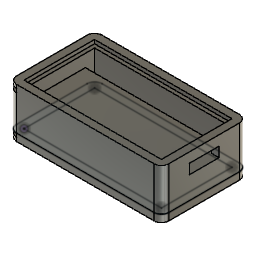
ESP 32 Case (Autodesk Fusion 360 design; units mm, degrees)
Autodesk Fusion 360 part; units mm, degrees
sketch "Sketch1" plane through (0, 0, 0) normal (0, 0, 1) x (1, 0, 0)
  line L0 (0, 0) -> (55.5, 0)
  line L1 (55.5, 0) -> (55.5, 28.5)
  line L2 (55.5, 28.5) -> (0, 28.5)
  line L3 (0, 28.5) -> (0, 0)
  line L4 (0, -3) -> (55.5, -3)
  line L5 (58.5, 0) -> (58.5, 28.5)
  line L6 (55.5, 31.5) -> (0, 31.5)
  line L7 (-3, 28.5) -> (-3, 0)
  arc A0 (58.5, 28.5) -> (55.5, 31.5) centre (55.5, 28.5) ccw
  arc A1 (55.5, -3) -> (58.5, 0) centre (55.5, 0) ccw
  arc A2 (-3, 0) -> (0, -3) centre (0, 0) ccw
  arc A3 (0, 31.5) -> (-3, 28.5) centre (0, 28.5) ccw
  dimension "d1" = 55.5
  dimension "d2" = 28.5
  dimension "d4" = 3
  dimension "d5" = 3
  dimension "d6" = 3
  dimension "d7" = 3
  constraint horizontal L0
  constraint vertical L1
  constraint horizontal L2
  constraint vertical L3
  constraint coincident L0.start L3.end
  constraint tangent L5 A0
  constraint tangent L6 A0
  constraint tangent L4 A1
  constraint tangent L5 A1
  constraint tangent L7 A2
  constraint tangent L4 A2
  constraint tangent L6 A3
  constraint tangent L7 A3
  measures "d1" distance of L0.start L0.end
  measures "d2" distance of L0.end L1.end
  measures "d4" radius of A0
  measures "d5" radius of A1
  measures "d6" radius of A2
  measures "d7" radius of A3
extrude "Extrude1" add sketch "Sketch1" along normal blind 12.7 makes body 1
extrude "Extrude2" add sketch "Sketch1" along normal blind 14 separate body makes body 2
sketch "Sketch3" plane through (0, 0, 0) normal (1, 0, 0) x (0, 1, 0)
  line L0 (0, 0) -> (28.5, 0)
  line L1 (28.5, 0) -> (28.5, 14)
  line L2 (28.5, 14) -> (0, 14)
  line L3 (0, 14) -> (0, 0)
  line L4 (13, 9) -> (28.5, 9)
  line L5 (28.5, 9) -> (28.5, 7)
  line L6 (28.5, 7) -> (13, 7)
  line L7 (13, 7) -> (0, 7)
  line L8 (0, 7) -> (0, 9)
  line L9 (0, 9) -> (13, 9)
  line L10 (3.75, 9) -> (3.75, 7)
  line L11 (24.75, 9) -> (24.75, 7)
  dimension "d13" = 5
  dimension "d14" = 5
  dimension "d15" = 2
  dimension "d16" = 21
  dimension "d17" = 3.75
  constraint horizontal L4
  constraint vertical L5
  constraint horizontal L6
  constraint coincident L1 L5.end
  constraint horizontal L7
  constraint vertical L8
  constraint horizontal L9
  constraint coincident L3 L8.end
  constraint coincident L9 L10.start
  constraint coincident L7 L10.end
  constraint perpendicular L7 L10
  constraint coincident L4 L11.start
  constraint coincident L6 L11.end
  constraint perpendicular L6 L11
  measures "d13" distance of L2 L9
  measures "d14" distance of L2 L4
  measures "d15" distance of L4 L6
  measures "d16" distance of L10 L11
  measures "d17" distance of L5 L11
extrude "Extrude3" add sketch "Sketch3" along normal blind 55.5 contours L4 L6 L7 L9 L10 L11 bodies 1 2
sketch "Sketch4" plane through (0, 0, 14) normal (0, 0, 1) x (-1, 0, 0)
  line L0 (0, 0) -> (0, -28.5)
  line L1 (0, -28.5) -> (-55.5, -28.5)
  line L2 (-55.5, -28.5) -> (-55.5, 0)
  line L3 (-55.5, 0) -> (0, 0)
  arc A0 (0, -31.5) -> (3, -28.5) centre (0, -28.5) ccw
  line L4 (3, -28.5) -> (3, 0)
  arc A1 (3, 0) -> (0, 3) centre (0, 0) ccw
  line L5 (0, 3) -> (-55.5, 3)
  arc A2 (-55.5, 3) -> (-58.5, 0) centre (-55.5, 0) ccw
  line L6 (-58.5, 0) -> (-58.5, -28.5)
  arc A3 (-58.5, -28.5) -> (-55.5, -31.5) centre (-55.5, -28.5) ccw
  line L7 (-55.5, -31.5) -> (0, -31.5)
  line L8 (-55.5, -31.5) -> (0, -31.5)
  line L9 (3, -28.5) -> (3, 0)
  line L10 (0, 3) -> (-55.5, 3)
  line L11 (-58.5, 0) -> (-58.5, -28.5)
  arc A4 (0, -31.5) -> (3, -28.5) centre (0, -28.5) ccw
  arc A5 (-58.5, -28.5) -> (-55.5, -31.5) centre (-55.5, -28.5) ccw
  arc A6 (-55.5, 3) -> (-58.5, 0) centre (-55.5, 0) ccw
  line L12 (1.5, -28.5) -> (1.5, 0)
  arc A7 (1.5, 0) -> (0, 1.5) centre (0, 0) ccw
  line L13 (0, 1.5) -> (-55.5, 1.5)
  arc A8 (-55.5, 1.5) -> (-57, 0) centre (-55.5, 0) ccw
  line L14 (-57, 0) -> (-57, -28.5)
  arc A9 (-57, -28.5) -> (-55.5, -30) centre (-55.5, -28.5) ccw
  line L15 (-55.5, -30) -> (0, -30)
  arc A10 (0, -30) -> (1.5, -28.5) centre (0, -28.5) ccw
  line L16 (0, 3) -> (0, 1.5)
  line L17 (0, -30) -> (0, -31.5)
  constraint coincident A3.end L7.start
  constraint coincident A0.start L7.end
  constraint coincident A0.end L4.start
  constraint coincident L4.end A1.start
  constraint coincident A1.end L5.start
  constraint coincident L5.end A2.start
  constraint coincident A2.end L6.start
  constraint coincident L6.end A3.start
  constraint concentric A6 A8
  constraint concentric A5 A9
  constraint concentric A4 A10
  constraint tangent L15 A10
  constraint tangent L12 A10
  constraint tangent A7 L13
  constraint tangent L12 A7
  constraint tangent L13 A8
  constraint tangent A8 L14
  constraint tangent L14 A9
  constraint tangent A9 L15
  constraint perpendicular L13 L16
  constraint perpendicular L8 L17
extrude "Extrude4" add sketch "Sketch4" along normal blind 1.5 contours L5 A2 L6 A3 L7 L8 L10 L11 A5 A6 L13 A8 L14 A9 L15 L16 L17 bodies 1
sketch "Sketch5" plane through (0, 0, 15.5) normal (0, 0, 1) x (-1, 0, 0)
  line L0 (0, 3) -> (-55.5, 3)
  arc A0 (-55.5, 3) -> (-58.5, 0) centre (-55.5, 0) ccw
  line L1 (-58.5, 0) -> (-58.5, -28.5)
  arc A1 (-58.5, -28.5) -> (-55.5, -31.5) centre (-55.5, -28.5) ccw
  line L2 (-55.5, -31.5) -> (0, -31.5)
  line L3 (0, -31.5) -> (0, -30)
  line L4 (0, -30) -> (-55.5, -30)
  arc A2 (-57, -28.5) -> (-55.5, -30) centre (-55.5, -28.5) ccw
  line L5 (-57, -28.5) -> (-57, 0)
  arc A3 (-55.5, 1.5) -> (-57, 0) centre (-55.5, 0) ccw
  line L6 (-55.5, 1.5) -> (0, 1.5)
  line L7 (0, 1.5) -> (0, 3)
  line L8 (-58.5, -28.5) -> (-58.5, 0)
  line L9 (-55.5, -31.5) -> (0, -31.5)
  line L10 (3, -28) -> (3, 0)
  arc A4 (3, 0) -> (0, 3) centre (0, 0) ccw
  arc A5 (0, -31.5) -> (3, -28) centre (0, -28.4643) ccw
  arc A6 (-58.5, -28.5) -> (-55.5, -31.5) centre (-55.5, -28.5) ccw
  arc A7 (-55.5, 3) -> (-58.5, 0) centre (-55.5, 0) ccw
  line L11 (0, 3) -> (-55.5, 3)
  line L12 (0, -28.4643) -> (0, 0)
  line L13 (0, 0) -> (-55.5, 0)
  line L14 (-55.5, 0) -> (-55.5, -28.5)
  line L15 (-55.5, -28.5) -> (0, -28.4643)
  constraint coincident L1.end A1.start
  constraint coincident A0.end L1.start
  constraint coincident A1.end L2.start
  constraint coincident L2.end L3.start
  constraint perpendicular L4 L10
  constraint tangent L0 A4
  constraint coincident L0.start L7.end
  constraint tangent L9 A5
  constraint coincident L0.end A0.start
  constraint coincident A5.centre L12.start
  constraint coincident A4.centre L12.end
  constraint coincident A0.centre A3.centre
  constraint perpendicular L12 L13
  constraint coincident A1.centre A2.centre
  constraint perpendicular L6 L14
extrude "Extrude5" add sketch "Sketch5" along normal blind 1.5 bodies 1
sketch "Sketch6" plane through (0, 0, 0) normal (0, 0, 1) x (1, 0, 0)
  line L0 (0, -3) -> (55.4843, -3)
  arc A0 (55.4843, -3) -> (58.5, 0) centre (55.4843, 0.0158) ccw
  arc A1 (58.5, 28.5) -> (55.4843, 31.4919) centre (55.5232, 28.5153) ccw
  line L1 (58.5, 28.5) -> (58.5, 0)
  line L2 (55.4843, 31.4919) -> (0, 31.4919)
  line L3 (0, -1.5) -> (55.4843, -1.5)
  arc A2 (55.4843, -1.5) -> (57, 0.0046) centre (55.4843, 0.0158) ccw
  line L4 (57, 28.5045) -> (57, 0.0046)
  arc A3 (57, 28.5045) -> (55.4958, 29.9919) centre (55.5232, 28.5153) ccw
  line L5 (55.4958, 29.9919) -> (0, 29.9919)
  line L6 (0, -1.5) -> (0, -3)
  line L7 (0, 29.9919) -> (0, 31.4919)
  constraint horizontal L0
  constraint tangent L0 A0
  constraint vertical L1
  constraint perpendicular L1 L2
  constraint perpendicular L0 L6
  constraint perpendicular L2 L7
  constraint concentric A0 A2
  constraint concentric A1 A3
  constraint tangent L3 A2
extrude "Extrude6" add sketch "Sketch6" against normal blind 1.5 bodies 1
sketch "Sketch7" plane through (0, 0, -1.5) normal (0, 0, -1) x (1, 0, 0)
  line L0 (57, -0.0046) -> (57, -28.5045)
  arc A0 (55.4958, -29.9919) -> (57, -28.5045) centre (55.5232, -28.5153) ccw
  line L1 (55.4958, -29.9919) -> (0, -29.9919)
  line L2 (0, -29.9919) -> (0, -31.4919)
  line L3 (0, -31.4919) -> (55.4843, -31.4919)
  arc A1 (55.4843, -31.4919) -> (58.5, -28.5) centre (55.5232, -28.5153) ccw
  line L4 (58.5, -28.5) -> (58.5, 0)
  arc A2 (58.5, 0) -> (55.4843, 3) centre (55.4843, -0.0158) ccw
  line L5 (55.4843, 3) -> (0, 3)
  line L6 (0, 3) -> (0, 1.5)
  line L7 (0, 1.5) -> (55.4843, 1.5)
  arc A3 (57, -0.0046) -> (55.4843, 1.5) centre (55.4843, -0.0158) ccw
  line L8 (55.4843, -31.4919) -> (0, -31.4919)
  line L9 (58.5, -28.5) -> (58.5, 0)
  line L10 (55.4843, 3) -> (0, 3)
  arc A4 (0, 3) -> (-3, 0) centre (0, 0) ccw
  line L11 (-3, 0) -> (-3, -28.5144)
  arc A5 (-3, -28.5144) -> (0, -31.4919) centre (0, -28.4918) ccw
  arc A6 (55.4843, -31.4919) -> (58.5, -28.5) centre (55.5232, -28.5153) ccw
  arc A7 (58.5, 0) -> (55.4843, 3) centre (55.4843, -0.0158) ccw
  line L12 (58.5, -28.5) -> (58.5, 0)
  line L13 (55.4843, -28.4919) -> (0, -28.4919)
  arc A8 (55.5, -28.4919) -> (55.4843, -28.4919) centre (55.4843, -31.4919) ccw
  line L14 (55.5, -28.4919) -> (55.5, -0.0146)
  arc A9 (55.5, -0.0146) -> (55.4843, 0) centre (55.4843, -0.0158) ccw
  line L15 (55.4843, 0) -> (0, 0)
  line L16 (0, 0) -> (0, -28.4919)
  dimension "d28" = -3
  constraint coincident L3.end A1.start
  constraint coincident L2.end L3.start
  constraint coincident A1.end L4.start
  constraint coincident L4.end A2.start
  constraint coincident A2.end L5.start
  constraint coincident L5.end L6.start
  constraint tangent A4 L11
  constraint perpendicular L1 L11
  constraint tangent L8 A5
extrude "Extrude7" add sketch "Sketch7" along normal blind 1.5 bodies 1
sketch "Sketch8" plane through (55.5, 0, 0) normal (-1, 0, 0) x (0, -1, 0)
  line L0 (-24.75, 9) -> (-3.75, 9)
  line L1 (-3.75, 9) -> (-3.75, 7)
  line L2 (-3.75, 7) -> (-24.75, 7)
  line L3 (-24.75, 7) -> (-24.75, 9)
  line L4 (-28.5, 0) -> (0, 0)
  line L5 (0, 0) -> (0, 14)
  line L6 (0, 14) -> (-28.5, 14)
  line L7 (-28.5, 14) -> (-28.5, 0)
  line L8 (-14.25, 9) -> (-20.25, 9)
  line L9 (-20.25, 9) -> (-20.25, 13)
  line L10 (-20.25, 13) -> (-14.25, 13)
  line L11 (-14.25, 13) -> (-14.25, 9)
  line L12 (-14.25, 13) -> (-8.25, 13)
  line L13 (-8.25, 13) -> (-8.25, 9)
  line L14 (-8.25, 9) -> (-14.25, 9)
  line L15 (-14.25, 9) -> (-14.25, 13)
  dimension "d31" = 6
  dimension "d32" = 4
  dimension "d33" = 6
  constraint horizontal L8
  constraint vertical L9
  constraint horizontal L10
  constraint vertical L11
  constraint midpoint L0 L8.start
  constraint horizontal L12
  constraint vertical L13
  constraint horizontal L14
  constraint vertical L15
  constraint coincident L0 L13.end
  measures "d31" distance of L9.end L10.end
  measures "d32" distance of L8.end L9.end
  measures "d33" distance of L10.end L12.end
extrude "Extrude8" cut sketch "Sketch8" against normal blind 10 contours L0 L8 L9 L10 L11 L15 | L0 L11 L12 L13 L14 L15 bodies 1
